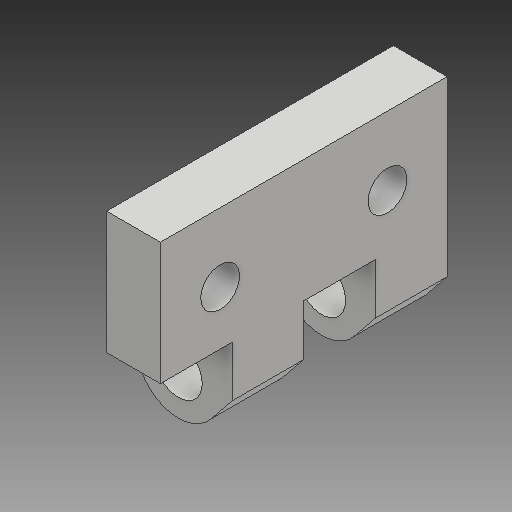
# Autodesk Inventor part: item_scharnier_2_teil
Saved by Autodesk Inventor 2018 (Build 220112000, 112)
## iProperties
Created: 2020-04-19
Part Number: item_scharnier_2_teil
Material: Generisch
Document SubType Name: Modeling
Designer: wepet
Density: 1 g/cm^3
Appearance: Vorgabe
Description: Scharnier für Aluprofil mit 2 Bohrungen (halbes Scharnier)
Mass: 0.011661 g
Surface Area: 0.542172 cm^2
Volume: 0.011661 cm^3
Author: wepet
Autodesk Inventor part; units mm, degrees
ref_plane "YZ Plane" through (0, 0, 0) normal (1, 0, 0) x (0, 1, 0)
ref_plane "XZ Plane" through (0, 0, 0) normal (0, 1, 0) x (-1, 0, 0)
ref_plane "XY Plane" through (0, 0, 0) normal (0, 0, 1) x (1, 0, 0)
sketch "Skizze1" plane through (0, 0, 0) normal (0, 1, 0) x (-1, 0, 0)
  line L0 (0, 0) -> (0.9, 0)
  line L1 (0.9, 0) -> (0.9, -2.9)
  line L2 (0.9, -2.9) -> (0, -2.9) construction
  line L3 (0, -2.9) -> (0, 0)
  circle A0 centre (0.9, -2.9) radius 0.4
  arc A1 (0.3556, -3.34) -> (0.9, -2.2) centre (0.9, -2.9) ccw
  line L4 (0, -2.9) -> (0.3556, -3.34)
  dimension "d0" = 0.9
  dimension "d2" = 0.8
  dimension "d3" = 1.4
  dimension "d4" = 2.9
  constraints: 10 end point, 2 centre point, 2 parallel, 2 point on circle, 1 coincident, 1 horizontal, 1 perpendicular, 1 point on line, 1 tangent
  measures "d0" distance of L1.end L2.end
  measures "d2" diameter of A0
  measures "d3" diameter of A1
  measures "d4" distance of L2.end L0.start
extrude "Extrusion1" add sketch "Skizze1" along normal blind 4.8
sketch "Skizze2" plane through (0, 0, 0) normal (1, 0, 0) x (0, 0, -1)
  line L0 (2.9, 0) -> (0, 0) construction
  line L1 (2.9, 0) -> (2.9, 4.8) construction
  line L2 (0, 4.8) -> (2.9, 4.8) construction
  line L3 (0, 0) -> (0, 4.8) construction
  line L4 (0, 4.8) -> (2.9, 4.8) construction
  line L5 (2.05, 4.8) -> (2.05, 0) construction
  line L6 (2.05, 0) -> (4.05, 0)
  line L7 (4.05, 0) -> (4.05, 1.2)
  line L8 (4.05, 1.2) -> (2.05, 1.2)
  line L9 (2.05, 1.2) -> (2.05, 0)
  line L10 (2.05, 3.6) -> (4.05, 3.6)
  line L11 (4.05, 3.6) -> (4.05, 2.4)
  line L12 (4.05, 2.4) -> (2.05, 2.4)
  line L13 (2.05, 2.4) -> (2.05, 3.6)
  dimension "d7" = 0.85
  dimension "d8" = 2
  dimension "d9" = 1.2
  dimension "d10" = 1.2
  dimension "d11" = 1.2
  constraints: 18 end point, 4 parallel, 4 point on line, 3 perpendicular, 2 horizontal
  measures "d7" distance between parallel lines of L1 L5
  measures "d8" distance of L8.end L7.end
  measures "d9" distance of L6.end L7.end
  measures "d10" distance of L10.end L11.end
  measures "d11" distance between parallel lines of L8 L12
extrude "Extrusion2" cut sketch "Skizze2" against normal blind 4
sketch "Skizze4" plane through (-0.9, 0, 0) normal (-1, 0, 0) x (0, 0, 1)
  line L0 (-2.05, 1.2) -> (-2.05, 0) construction
  line L1 (0, 0) -> (-2.05, 0) construction
  line L2 (0, 0) -> (0, 4.8) construction
  line L3 (-2.2, 4.8) -> (0, 4.8) construction
  line L4 (-2.2, 3.6) -> (-2.2, 4.8) construction
  line L5 (-2.2, 3.6) -> (-2.05, 3.6) construction
  line L6 (-2.05, 3.6) -> (-2.05, 2.4) construction
  line L7 (-2.05, 2.4) -> (-2.2, 2.4) construction
  line L8 (-2.2, 1.2) -> (-2.2, 2.4) construction
  line L9 (-2.2, 1.2) -> (-2.05, 1.2) construction
  line L10 (0, 0) -> (0, 4.8) construction
  line L11 (-1.15, 3.8) -> (-1.15, 1) construction
  line L12 (0, 2.4) -> (-2.05, 2.4) construction
  point P0 (-1.15, 2.4)
  dimension "d30" = 2.8
  dimension "d31" = 1.15
  constraints: 4 end point, 2 midpoint, 1 perpendicular, 1 point on line, 1 vertical
  measures "d30" distance of L11.start L11.end
  measures "d31" distance between parallel lines of L2 L11
hole "Bohrung2" at (-0.9, 3.8, -1.15) at (-0.9, 1, -1.15) direction (1, 0, 0) diameter 0.65 end through all countersink diameter 1 countersink angle 90
